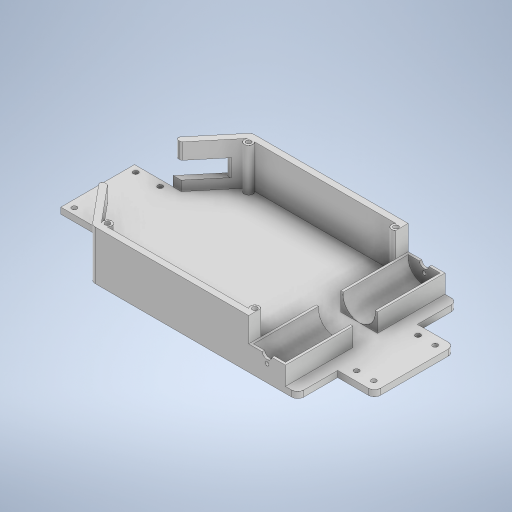
# Autodesk Inventor part: Pieza4
Saved by Autodesk Inventor 2024.3 (Build 283343000, 343)
## iProperties
Created: 2025-02-01
Part Number: Pieza4
Material: Genérico
Document SubType Name: Modeling
Designer: Jorge
Density: 1 g/cm^3
Appearance: Valor por defecto
Author: Jorge
Autodesk Inventor part; units mm, degrees
sketch "Boceto1" plane through (0, 0, 0) normal (0, 1, 0) x (-1, 0, 0)
  line L0 (197.3419, -130) -> (35, -130)
  line L1 (5, -32.5) -> (30, -32.5)
  line L2 (30, -32.5) -> (30, -97.5)
  line L3 (30, -97.5) -> (5, -97.5)
  line L4 (30, -5) -> (30, -32.5)
  line L5 (30, -97.5) -> (30, -125)
  line L6 (0, -37.5) -> (0, -92.5)
  arc A0 (5, -32.5) -> (0, -37.5) centre (5, -37.5) ccw
  arc A1 (0, -92.5) -> (5, -97.5) centre (5, -92.5) ccw
  line L7 (35, 0) -> (40, 0) construction
  line L8 (40, 0) -> (40, -130) construction
  line L9 (40, -130) -> (70, -130)
  line L10 (70, -130) -> (70, -75)
  line L11 (70, -75) -> (40, -75)
  line L12 (40, -75) -> (40, -130)
  line L13 (40, 0) -> (70, 0)
  line L14 (70, 0) -> (70, -55)
  line L15 (70, -55) -> (40, -55)
  line L16 (40, -55) -> (40, 0)
  arc A2 (30, -125) -> (35, -130) centre (35, -125) ccw
  arc A3 (35, 0) -> (30, -5) centre (35, -5) ccw
  line L17 (70, 0) -> (70, -5) construction
  line L18 (70, -130) -> (70, -125) construction
  line L19 (70, -125) -> (195, -125)
  line L20 (70, -5) -> (195, -5)
  line L21 (195, -5) -> (220, -5) construction
  line L22 (220, -5) -> (220, -125) construction
  line L23 (220, -125) -> (195, -125) construction
  line L24 (0, -65) -> (285, -65) construction
  line L25 (220, -65) -> (220, -95) construction
  line L26 (220, -65) -> (220, -35) construction
  line L27 (220, -35) -> (255, -35) construction
  line L28 (255, -35) -> (255, -95) construction
  line L29 (255, -95) -> (220, -95) construction
  line L30 (195, -5) -> (220, -35)
  line L31 (195, -125) -> (220, -95)
  line L32 (220, -95) -> (255, -95)
  line L33 (220, -35) -> (255, -35)
  line L34 (255, -35) -> (255, -95)
  line L35 (207.5, -110) -> (211.3411, -113.2009) construction
  line L36 (197.3419, -130) -> (226.5085, -95)
  line L37 (197.3419, 0) -> (226.5085, -35)
  line L38 (70, 0) -> (197.3419, 0)
  line L39 (35, 0) -> (40, 0)
  line L40 (255, -95) -> (258, -95)
  line L41 (258, -95) -> (258, -35)
  line L42 (258, -35) -> (255, -35)
  line L43 (255, -35) -> (255, -95)
  point P0 (0, 0)
  point P1 (30, -130)
  dimension "d5" = 5
  dimension "d7" = 30
  dimension "d8" = 55
  dimension "d9" = 55
  dimension "d10" = 5
  dimension "d11" = 5
  dimension "d12" = 125
  dimension "d13" = 25
  dimension "d14" = 30
  dimension "d15" = 30
  dimension "d16" = 35
  dimension "d17" = 5
  dimension "d62" = 3
  constraints: 88 end point, 11 perpendicular, 11 point on line, 8 parallel, 8 point on circle, 8 tangent, 5 horizontal, 4 centre point, 3 collinear, 3 midpoint, 2 equal radius, 2 symmetric about line, 2 vertical
  measures "d5" radius of A0
  measures "d7" distance of L11.end L10.end
  measures "d8" distance of L10.end L9.end
  measures "d9" distance of L13.end L14.end
  measures "d10" radius of A2
  measures "d11" distance of L13.end L17.end
  measures "d12" distance of L18.end L19.end
  measures "d13" distance of L20.end L21.end
  measures "d14" distance of L25.start L25.end
  measures "d15" distance of L25.start L26.end
  measures "d16" distance of L26.end L27.end
  measures "d17" distance of L35.start L35.end
  measures "d62" distance of L42.end L41.end
extrude "Extrusión1" add sketch "Boceto1" along normal blind 40 contours L0 L10 L19 L31 L32 L36 | L33 L30 L20 L14 L38 L37
extrude "Extrusión2" add sketch "Boceto1" along normal blind 5 contours L32 L31 L19 L10 L11 L12 L0 A2 L5 L2 L4 A3 L39 L16 L15 L14 L20 L30 L33 L34 | L34 L42 L41 L40 | L3 A1 L6 A0 L1 L2
extrude "Extrusión3" add sketch "Boceto1" along normal blind 20 contours L0 L12 L11 L10 | L14 L15 L16 L13
fillet "Empalme1" radius 5 2 edges at (-197.3419, 20, 0) (-197.3419, 20, -130)
ref_plane "Plano de trabajo1" through (0, 0, -65) normal (0, 0, 1) x (1, 0, 0)
sketch "Boceto2" plane through (0, 0, -65) normal (0, 0, 1) x (1, 0, 0)
  line L0 (-40, 20) -> (-70, 20) construction
  line L1 (-70, 20) -> (-68, 20) construction
  line L2 (-40, 5) -> (-40, 20) construction
  line L3 (-40, 20) -> (-42, 20) construction
  arc A0 (-68, 20) -> (-42, 20) centre (-55, 18.1333) ccw
  line L4 (-68, 20) -> (-68, 21.6532)
  line L5 (-68, 21.6532) -> (-42, 21.6532)
  line L6 (-42, 21.6532) -> (-42, 20)
  point P0 (0, 0)
  dimension "d26" = 2
  dimension "d27" = 2
  constraints: 10 end point, 2 perpendicular, 2 point on circle, 2 point on line, 1 centre point, 1 vertical
  measures "d26" distance of L0.end L1.end
  measures "d27" distance of L0.start L3.end
extrude "Extrusión4" cut sketch "Boceto2" along normal mid plane 126
sketch "Boceto3" plane through (0, 0, -65) normal (0, 0, 1) x (1, 0, 0)
  line L0 (-68, 20) -> (-42, 20) construction
  line L1 (-55, 20) -> (-59, 20) construction
  line L2 (-55, 20) -> (-51, 20) construction
  line L3 (-55, 20) -> (-55, 16.5) construction
  arc A0 (-59, 20) -> (-51, 20) centre (-55, 20.5357) ccw
  arc A1 (-51, 20) -> (-59, 20) centre (-55, 15.3068) ccw
  point P0 (0, 0)
  dimension "d30" = 4
  dimension "d33" = 3.5
  constraints: 6 end point, 5 point on circle, 2 centre point, 2 point on line, 1 midpoint, 1 perpendicular
  measures "d30" distance of L1.start L1.end
  measures "d33" distance of L1.start L3.end
extrude "Extrusión5" cut sketch "Boceto3" along normal through all both and the other way through all
sketch "Boceto4" plane through (0, 0, -65) normal (0, 0, 1) x (1, 0, 0)
  arc A0 (-59, 20) -> (-51, 20) centre (-55, 20.5357) ccw construction
  line L0 (-55, 16.5) -> (-55, 13.5) construction
  circle A1 centre (-55, 13.5) radius 1.5
  point P0 (0, 0)
  dimension "d36" = 3
  dimension "d37" = 3
  constraints: 2 end point, 1 centre point, 1 coincident, 1 point on circle, 1 vertical
  measures "d36" distance of L0.start L0.end
  measures "d37" diameter of A1
extrude "Extrusión6" cut sketch "Boceto4" along normal through all both and the other way through all
sketch "Boceto5" plane through (0, 5, 0) normal (0, 1, 0) x (1, 0, 0)
  line L0 (-30, 97.5) -> (-30, 125) construction
  line L1 (-30, 32.5) -> (-30, 97.5) construction
  line L2 (0, 37.5) -> (0, 92.5) construction
  line L3 (0, 65) -> (-30, 65) construction
  line L4 (0, 97.5) -> (-15, 97.5) construction
  line L5 (-5, 97.5) -> (-30, 97.5) construction
  line L6 (-15, 97.5) -> (-15, 32.5) construction
  line L7 (-30, 32.5) -> (-5, 32.5) construction
  line L8 (-15, 65) -> (-15, 40) construction
  line L9 (-15, 40) -> (-20, 40) construction
  line L10 (-20, 40) -> (-22, 40) construction
  circle A0 centre (-22, 40) radius 2
  circle A1 centre (-8, 40) radius 2
  circle A2 centre (-22, 90) radius 2
  circle A3 centre (-8, 90) radius 2
  point P0 (0, 0)
  dimension "d40" = 15
  dimension "d41" = 25
  dimension "d42" = 5
  dimension "d43" = 2
  constraints: 14 end point, 3 centre point, 3 midpoint, 3 point on line, 3 symmetric about line, 2 perpendicular, 1 coincident, 1 horizontal, 1 horizontal alignment, 1 vertical, 5 other
  measures "d40" distance of L4.start L4.end
  measures "d41" distance of L8.start L8.end
  measures "d42" distance of L8.end L9.end
  measures "d43" distance of L9.end L10.end
extrude "Extrusión7" cut sketch "Boceto5" against normal blind 10
sketch "Boceto6" plane through (0, 5, 0) normal (0, 1, 0) x (1, 0, 0)
  line L0 (-70, 55) -> (-70, 5) construction
  line L1 (-70, 5) -> (-70, 10) construction
  line L2 (-70, 10) -> (-75, 10) construction
  line L3 (-75, 10) -> (-75, 5) construction
  line L4 (-75, 5) -> (-70, 10) construction
  line L5 (-75, 10) -> (-70, 5) construction
  circle A0 centre (-72.5, 7.5) radius 2
  arc A1 (-70, 10) -> (-75, 5) centre (-72.5, 7.5) ccw
  line L6 (-70, 0) -> (-70, 5) projected
  line L7 (-70, 10) -> (-70, 5)
  line L8 (-70, 5) -> (-75, 5)
  line L9 (0, 37.5) -> (0, 92.5) construction
  line L10 (0, 65) -> (-255, 65) construction
  line L11 (-255, 95) -> (-255, 35) construction
  line L12 (0, 65) -> (-127.5, 65) construction
  line L13 (-127.5, 65) -> (-127.5, 0) construction
  line L14 (-195, 0) -> (-35, 0) construction
  line L15 (-70, 125) -> (-70, 120) construction
  circle A2 centre (-72.5, 122.5) radius 2
  arc A3 (-75, 125) -> (-70, 120) centre (-72.5, 122.5) ccw
  line L16 (-70, 120) -> (-70, 125)
  line L17 (-70, 125) -> (-75, 125)
  line L18 (-195, 5) -> (-220, 35) construction
  line L19 (-195, 125) -> (-70, 125) construction
  line L20 (-195, 5) -> (-195, 125) construction
  line L21 (-70, 65) -> (-132.5, 65) construction
  line L22 (-132.5, 65) -> (-132.5, 130) construction
  line L23 (-35, 130) -> (-195, 130) construction
  circle A4 centre (-192.5, 7.5) radius 2
  arc A5 (-190, 5) -> (-195, 10) centre (-192.5, 7.5) ccw
  line L24 (-195, 10) -> (-195, 5)
  line L25 (-195, 5) -> (-190, 5)
  arc A6 (-195, 120) -> (-190, 125) centre (-192.5, 122.5) ccw
  circle A7 centre (-192.5, 122.5) radius 2
  line L26 (-195, 125) -> (-190, 125)
  line L27 (-195, 120) -> (-195, 125)
  arc A8 (-195, 125) -> (-192.5, 118.9645) centre (-192.5, 122.5) ccw
  line L28 (-190, 125) -> (-195, 125)
  arc A9 (-192.5, 11.0355) -> (-195, 5) centre (-192.5, 7.5) ccw
  point P0 (0, 0)
  point P1 (-195, 120)
  dimension "d47" = 5
  dimension "d48" = 4
  dimension "d49" = 127.5
  dimension "d50" = 62.5
  constraints: 42 end point, 15 point on circle, 13 symmetric about line, 10 centre point, 5 perpendicular, 5 point on line, 4 midpoint, 2 coincident, 2 vertical, 1 collinear, 6 other
  measures "d47" distance of L1.end L2.end
  measures "d48" diameter of A0
  measures "d49" distance of L10.start L12.end
  measures "d50" distance of L21.start L21.end
extrude "Extrusión8" add sketch "Boceto6" along normal blind 35
extrude "Extrusión9" cut sketch "Boceto6" against normal blind 35 contours A0 | A2 | A4 | A7
sketch "Boceto7" plane through (0, 5, 0) normal (0, 1, 0) x (1, 0, 0)
  line L0 (-255, 35) -> (-226.5085, 35) construction
  line L1 (-198.8411, 128.2009) -> (-226.5085, 95) construction
  line L2 (-226.5085, 35) -> (-226.5085, 95) construction
  line L3 (-226.5085, 65) -> (-255, 65) construction
  line L4 (-255, 95) -> (-255, 35) construction
  line L5 (-226.5085, 95) -> (-255, 95) construction
  line L6 (-240.7543, 95) -> (-240.7543, 35) construction
  line L7 (-226.5085, 35) -> (-229.5085, 35) construction
  circle A0 centre (-252, 40) radius 2
  circle A1 centre (-252, 90) radius 2
  line L8 (-226.5085, 35) -> (-226.5085, 40) construction
  line L9 (-226.5085, 40) -> (-232.0085, 40) construction
  circle A2 centre (-232.0085, 40) radius 2
  circle A3 centre (-232.0085, 90) radius 2
  point P0 (0, 0)
  dimension "d64" = 5.5
  dimension "d65" = 4
  constraints: 12 end point, 4 centre point, 4 midpoint, 2 coincident, 2 point on line, 2 symmetric about line, 1 horizontal, 1 vertical, 2 other
  measures "d64" distance of L9.start L9.end
  measures "d65" diameter of A2
extrude "Extrusión10" cut sketch "Boceto7" against normal blind 35
ref_plane "Plano de trabajo2" through (0, 0, -65) normal (0, 0, 1) x (1, 0, 0)
ref_plane "Plano de trabajo3" through (0, 0, -65) normal (0, 0, 1) x (1, 0, 0)
sketch "Boceto9" plane through (0, 0, -65) normal (0, 0, 1) x (1, 0, 0)
  line L0 (-226.5085, 5) -> (-226.5085, 40) construction
  line L1 (-226.5085, 22.5) -> (-226.5085, 27)
  line L2 (-226.5085, 27) -> (-204.8867, 27)
  line L3 (-204.8867, 27) -> (-204.8867, 13)
  line L4 (-204.8867, 13) -> (-226.5085, 13)
  line L5 (-226.5085, 13) -> (-226.5085, 27)
  point P0 (0, 0)
  dimension "d79" = 4.5
  dimension "d80" = 14
  constraints: 10 end point, 2 parallel, 1 horizontal, 1 midpoint, 1 perpendicular, 1 point on line
  measures "d79" distance of L1.start L1.end
  measures "d80" distance of L2.end L3.end
extrude "Extrusión12" cut sketch "Boceto9" along normal through all both and the other way through all
fillet "Empalme2" radius 2 8 edges at (-204.8867, 20, -16.864) (-204.8867, 20, -9.0538) (-204.8867, 20, -120.9462) (-204.8867, 20, -113.136) (-220, 33.5, -35) (-226.5085, 33.5, -35) (-226.5085, 33.5, -95) (-220, 33.5, -95)
